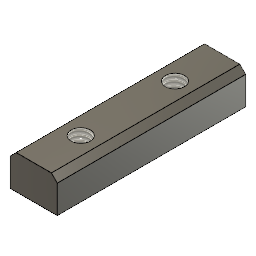
Screw Plate v1 (Autodesk Fusion 360 design; units mm, degrees)
Autodesk Fusion 360 part; units mm, degrees
sketch "Sketch1" plane through (0, 0, 0) normal (0, 1, 0) x (1, 0, 0)
  line L0 (2, -8) -> (-2, -8)
  line L1 (-2, -8) -> (-2, 8)
  line L2 (-2, 8) -> (2, 8)
  line L3 (2, 8) -> (2, -8)
  line L4 (0, 3.9919) -> (0, -4.0081) construction
  circle A0 centre (0, 3.9919) radius 1
  circle A1 centre (0, -4.0081) radius 1
  dimension "d1" = 16
  dimension "d2" = 4
  dimension "d3" = 8
  dimension "d4" = 2
  dimension "d5" = 2
  measures "d4" diameter of A0
  measures "d5" diameter of A1
extrude "Extrude1" add sketch "Sketch1" along normal blind 2.9
chamfer "Chamfer1" distance 0.5 angle 45 1 edges at (2, 2.9, 0)
chamfer "Chamfer2" distance 0.5 angle 45 1 edges at (-2, 2.9, 0)
thread "Thread1" "ISO Metric profile 2.0 M2x0.4 6H" major diameter 2.074 minor diameter 1.623 pitch 0.4 angle 60 resizes the face on face at (0.9988, 1.9333, 4.058)
thread "Thread2" "ISO Metric profile 2.0 M2x0.4 6H" major diameter 2.074 minor diameter 1.623 pitch 0.4 angle 60 resizes the face on face at (0.9988, 0.9667, -4.0417)
